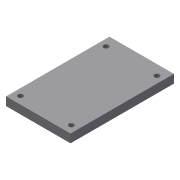
# Autodesk Inventor part: arm_1_case
Saved by Autodesk Inventor 2018 (Build 220112000, 112)
## iProperties
Created: 2018-02-11
Part Number: arm_1_case
Material: Generic
Document SubType Name: Modeling
Designer: Bardo91
Density: 1 g/cm^3
Appearance: Default
Author: Bardo91
Autodesk Inventor part; units mm, degrees
ref_plane "YZ Plane" through (0, 0, 0) normal (1, 0, 0) x (0, 1, 0)
ref_plane "XZ Plane" through (0, 0, 0) normal (0, 1, 0) x (-1, 0, 0)
ref_plane "XY Plane" through (0, 0, 0) normal (0, 0, 1) x (1, 0, 0)
sketch "Sketch1" plane through (0, 0, 0) normal (0, 0, 1) x (1, 0, 0)
  line L0 (0, 0) -> (38, 0)
  line L1 (38, 0) -> (38, 61)
  line L2 (38, 61) -> (0, 61)
  line L3 (0, 61) -> (0, 0)
  line L4 (0, 61) -> (4, 61)
  line L5 (4, 61) -> (4, 55)
  line L6 (38, 61) -> (34, 61)
  line L7 (34, 61) -> (34, 55)
  line L8 (38, 0) -> (34, 0)
  line L9 (34, 0) -> (34, 4.5)
  line L10 (0, 0) -> (4, 0)
  line L11 (4, 0) -> (4, 4.5)
  circle A0 centre (4, 4.5) radius 1.5
  circle A1 centre (34, 4.5) radius 1.5
  circle A2 centre (34, 55) radius 1.5
  circle A3 centre (4, 55) radius 1.5
  dimension "d0" = 38
  dimension "d1" = 61
  dimension "d2" = 4
  dimension "d3" = 6
  dimension "d4" = 4
  dimension "d5" = 6
  dimension "d6" = 4
  dimension "d7" = 4.5
  dimension "d8" = 4
  dimension "d9" = 4.5
  dimension "d10" = 3
  dimension "d11" = 3
  dimension "d12" = 3
  dimension "d13" = 3
  constraints: 24 end point, 7 perpendicular, 4 centre point, 4 coincident, 4 point on line, 1 horizontal
  measures "d0" distance of L0.start L0.end
  measures "d1" distance of L0.end L1.end
  measures "d2" distance of L2.end L4.end
  measures "d3" distance of L4.end L5.end
  measures "d4" distance of L1.end L6.end
  measures "d5" distance of L6.end L7.end
  measures "d6" distance of L0.end L8.end
  measures "d7" distance of L8.end L9.end
  measures "d8" distance of L0.start L10.end
  measures "d9" distance of L10.end L11.end
  measures "d10" diameter of A0
  measures "d11" diameter of A1
  measures "d12" diameter of A2
  measures "d13" diameter of A3
extrude "Extrusion1" add sketch "Sketch1" along normal blind 5
body "Solid1"
